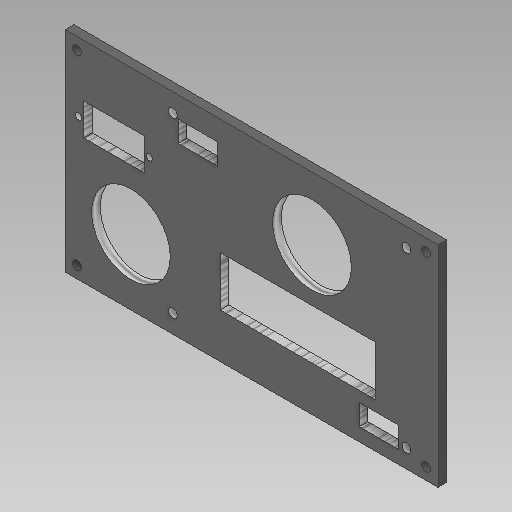
# Autodesk Inventor part: 基本板上
Saved by Autodesk Inventor 2017 (Build 210142000, 142)
## iProperties
Part Number: 基本板上
Material: アルミニウム 5052
Document SubType Name: Modeling
Designer: HISAAKI
Density: 2.68 g/cm^3
Appearance: サテン - ブラシ仕上げ 重厚
Mass: 72.7242 g
Surface Area: 199.157 cm^2
Volume: 27.1359 cm^3
Author: HISAAKI
Autodesk Inventor part; units mm, degrees
ref_plane "YZ Plane" through (0, 0, 0) normal (1, 0, 0) x (0, 1, 0)
ref_plane "XZ Plane" through (0, 0, 0) normal (0, 1, 0) x (-1, 0, 0)
ref_plane "XY Plane" through (0, 0, 0) normal (0, 0, 1) x (1, 0, 0)
sketch "スケッチ1" plane through (0, 0, 0) normal (0, 0, 1) x (1, 0, 0)
  line L0 (0, 0) -> (142, 0)
  line L1 (142, 0) -> (142, 80)
  line L2 (142, 80) -> (0, 80)
  line L3 (0, 80) -> (0, 0)
  dimension "d40" = 142
  dimension "d41" = 80
  constraints: 8 end point, 2 parallel, 1 horizontal, 1 perpendicular
  measures "d40" distance of L2.end L1.end
  measures "d41" distance of L1.end L0.end
extrude "押し出し1" add sketch "スケッチ1" along normal blind 3.3
hole "穴5" at (4.5, 75.5, 3.3) direction (0, 0, -1) diameter 3.4 end through all
hole "穴6" at (137.5, 75.5, 3.3) direction (0, 0, -1) diameter 3.4 end through all
hole "穴7" at (137.5, 4.5, 3.3) direction (0, 0, -1) diameter 3.4 end through all
hole "穴8" at (4.5, 4.5, 3.3) direction (0, 0, -1) diameter 3.4 end through all
hole "穴9" at (130, 73, 3.3) direction (0, 0, -1) diameter 3.4 end through all
hole "穴10" at (130, 7, 3.3) direction (0, 0, -1) diameter 3.4 end through all
hole "穴13" at (41, 73, 3.3) direction (0, 0, -1) diameter 3.4 end through all
hole "穴14" at (41, 7, 3.3) direction (0, 0, -1) diameter 3.4 end through all
sketch "スケッチ2" plane through (0, 0, 3.3) normal (0, 0, 1) x (1, 0, 0)
  line L0 (7, 60) -> (30, 60)
  line L1 (30, 60) -> (30, 47.8)
  line L2 (30, 47.8) -> (7, 47.8)
  line L3 (7, 47.8) -> (7, 60)
  point P0 (0, 0)
  dimension "d132" = 23
  dimension "d133" = 12.2
  constraints: 8 end point, 2 parallel, 1 horizontal, 1 perpendicular
  measures "d132" distance of L1.end L2.end
  measures "d133" distance of L0.end L1.end
extrude "押し出し2" cut sketch "スケッチ2" against normal blind 10
hole "穴15" at (5, 53.9, 3.3) direction (0, 0, -1) diameter 2.4 end through all
hole "穴16" at (32, 53.9, 3.3) direction (0, 0, -1) diameter 2.4 end through all
sketch "スケッチ5" plane through (0, 0, 3.3) normal (0, 0, 1) x (1, 0, 0)
  line L0 (142, 0) -> (142, 80) projected
  line L1 (142, 0) -> (142, 5)
  line L2 (142, 5) -> (127, 5)
  line L3 (127, 5) -> (127, 13)
  line L4 (127, 13) -> (112, 13)
  line L5 (112, 13) -> (112, 5)
  line L6 (112, 5) -> (127, 5)
  line L7 (142, 0) -> (142, 17)
  line L8 (142, 17) -> (118, 17)
  line L9 (118, 17) -> (118, 36)
  line L10 (118, 36) -> (59, 36)
  line L11 (59, 36) -> (59, 17)
  line L12 (59, 17) -> (118, 17)
  line L13 (142, 80) -> (0, 80) projected
  line L14 (0, 80) -> (43, 80)
  line L15 (43, 80) -> (43, 72)
  line L16 (43, 72) -> (58, 72)
  line L17 (58, 72) -> (58, 64)
  line L18 (58, 64) -> (43, 64)
  line L19 (43, 64) -> (43, 72)
  point P0 (0, 0)
  dimension "d171" = 5
  dimension "d172" = 15
  dimension "d173" = 8
  dimension "d174" = 15
  dimension "d175" = 17
  dimension "d176" = 24
  dimension "d177" = 19
  dimension "d178" = 59
  dimension "d179" = 43
  dimension "d180" = 8
  dimension "d181" = 15
  dimension "d182" = 8
  constraints: 36 end point, 14 perpendicular, 5 point on line, 1 horizontal
  measures "d171" distance of L0.start L1.end
  measures "d172" distance of L1.end L2.end
  measures "d173" distance of L2.end L3.end
  measures "d174" distance of L3.end L4.end
  measures "d175" distance of L0.start L7.end
  measures "d176" distance of L7.end L8.end
  measures "d177" distance of L8.end L9.end
  measures "d178" distance of L9.end L10.end
  measures "d179" distance of L13.end L14.end
  measures "d180" distance of L14.end L15.end
  measures "d181" distance of L15.end L16.end
  measures "d182" distance of L16.end L17.end
extrude "押し出し4" cut sketch "スケッチ5" against normal blind 10
sketch "スケッチ6" plane through (0, 0, 3.3) normal (0, 0, 1) x (1, 0, 0)
  line L0 (59, 36) -> (118, 36) projected
  line L1 (59, 36) -> (59, 56)
  line L2 (59, 56) -> (94, 56)
  circle A0 centre (94, 56) radius 15
  point P0 (0, 0)
  dimension "d185" = 20
  dimension "d187" = 35
  dimension "d188" = 30
  constraints: 4 end point, 1 centre point, 1 coincident, 1 horizontal, 1 vertical
  measures "d185" distance of L0.start L1.end
  measures "d187" distance of L1.end L2.end
  measures "d188" diameter of A0
extrude "押し出し5" cut sketch "スケッチ6" against normal blind 10
sketch "スケッチ7" plane through (0, 0, 3.3) normal (0, 0, 1) x (1, 0, 0)
  circle A0 centre (25, 25) radius 15
  point P0 (0, 0)
  dimension "d191" = 30
  constraints: 1 centre point
  measures "d191" diameter of A0
extrude "押し出し6" cut sketch "スケッチ7" against normal blind 10
